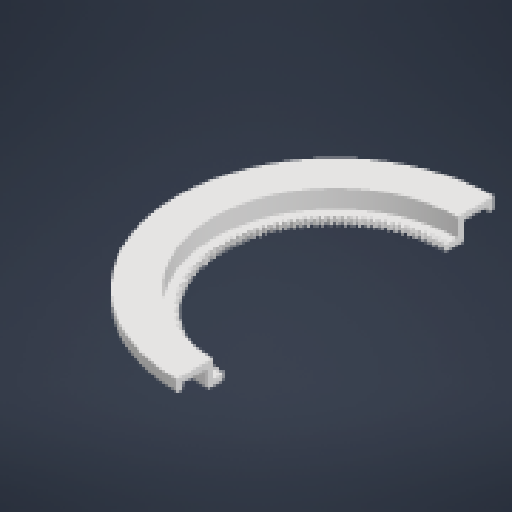
# Autodesk Inventor part: outerspinnerV3
Saved by Autodesk Inventor 2026 (Build 300175050, 175E)
## iProperties
Created: 2026-03-26
Part Number: outerspinnerV3
Material: Generic
Document SubType Name: Modeling
Designer: sniel
Density: 1 g/cm^3
Appearance: Default
Author: sniel
Autodesk Inventor part; units mm, degrees
ref_plane "YZ Plane" through (0, 0, 0) normal (1, 0, 0) x (0, 1, 0)
ref_plane "XZ Plane" through (0, 0, 0) normal (0, 1, 0) x (-1, 0, 0)
ref_plane "XY Plane" through (0, 0, 0) normal (0, 0, 1) x (1, 0, 0)
sketch "Sketch1" plane through (0, 0, 0) normal (0, 0, 1) x (1, 0, 0)
  line L0 (0, 0) -> (-100, 0)
  line L1 (-100, 0) -> (-100, 20)
  line L2 (-100, 20) -> (-130, 20)
  line L3 (-130, 20) -> (-130, 0)
  line L4 (-130, 0) -> (-100, 0)
  line L5 (-130, 0) -> (-125, 0)
  line L6 (-125, 0) -> (-125, 15)
  line L7 (-100, 0) -> (-105, 0)
  line L8 (-105, 0) -> (-105, 15)
  line L9 (-105, 15) -> (-125, 15)
  line L10 (0, -4) -> (0, 24) projected
  line L11 (-125, 15) -> (-125, 10)
  line L12 (-125, 10) -> (-130, 10)
  line L13 (-125, 15) -> (-115, 15)
  line L14 (-115, 15) -> (-117, 15)
  line L15 (-117, 15) -> (-117, 11)
  line L16 (-117, 11) -> (-113, 11)
  line L17 (-113, 11) -> (-113, 15)
  line L18 (-117, 15) -> (-119, 15)
  line L19 (-119, 15) -> (-119, 13)
  line L20 (-119, 13) -> (-117, 13)
  line L21 (-113, 15) -> (-111, 15)
  line L22 (-111, 15) -> (-111, 13)
  line L23 (-111, 13) -> (-113, 13)
  line L24 (-119, 15) -> (-118, 15)
  line L25 (-118, 15) -> (-118, 14)
  line L26 (-118, 14) -> (-119, 14)
  line L27 (-119, 14) -> (-119, 15)
  line L28 (-111, 15) -> (-112, 15)
  line L29 (-112, 15) -> (-112, 14)
  line L30 (-112, 14) -> (-111, 14)
  line L31 (-111, 14) -> (-111, 15)
  line L32 (-117, 13) -> (-119, 13)
  line L33 (-119, 13) -> (-119, 11)
  line L34 (-119, 11) -> (-117, 11)
  line L35 (-117, 11) -> (-117, 13)
  line L36 (-113, 13) -> (-111, 13)
  line L37 (-111, 13) -> (-111, 11)
  line L38 (-111, 11) -> (-113, 11)
  line L39 (-113, 11) -> (-113, 13)
  line L40 (-118, 14) -> (-112, 14)
  line L41 (-118, 14) -> (-118, 13)
  line L42 (-112, 14) -> (-112, 13)
  dimension "d0" = 100
  dimension "d1" = 20
  dimension "d2" = 30
  dimension "d3" = 5
  dimension "d4" = 15
  dimension "d5" = 5
  dimension "d7" = 5
  dimension "d8" = 2
  dimension "d9" = 4
  dimension "d10" = 4
  dimension "d11" = 2
  dimension "d12" = 2
  dimension "d13" = 2
  dimension "d22" = 1
  dimension "d23" = 1
  dimension "d24" = 1
  constraints: 84 end point, 16 perpendicular, 10 point on line, 8 parallel, 6 midpoint, 5 horizontal
  measures "d0" distance of L0.start L0.end
  measures "d1" distance of L0.end L1.end
  measures "d2" distance of L1.end L2.end
  measures "d3" distance of L3.end L5.end
  measures "d4" distance of L5.end L6.end
  measures "d5" distance of L0.end L7.end
  measures "d7" distance of L6.end L11.end
  measures "d8" distance of L13.end L14.end
  measures "d9" distance of L14.end L15.end
  measures "d10" distance of L15.end L16.end
  measures "d11" distance of L14.end L18.end
  measures "d12" distance of L18.end L19.end
  measures "d13" distance of L17.end L21.end
  measures "d22" distance of L24.end L25.end
  measures "d23" distance of L30.end L29.end
  measures "d24" distance of L29.end L28.end
revolve "Revolution1" add sketch "Sketch1" angle 360 about axis through (0, -10, 0) along (0, 1, 0) contours L4 L8 L9 L6 L12 L3 L2 L1 | L22 L30 L29 L9 | L9 L25 L26 L19
sketch "Sketch3" plane through (0, 0, 0) normal (0, -1, 0) x (1, 0, 0)
  circle A0 centre (0, 0) radius 102.0421
  arc A1 (-3.6556, 92.7167) -> (-4.7504, 92.6747) centre (-0.6449, 0) ccw
  arc A2 (-2.5377, 89.8188) -> (-3.6556, 92.7167) centre (-21.6763, 84.1004) ccw
  arc A3 (-2.4763, 89.6815) -> (-2.5377, 89.8188) centre (-14.4025, 84.4303) ccw
  arc A4 (-1.4378, 89.6967) -> (-2.4763, 89.6815) centre (-0.6449, 0) ccw
  arc A5 (-0.3693, 92.7652) -> (-1.4378, 89.6967) centre (17.8975, 84.684) ccw
  arc A6 (0.7262, 92.7554) -> (-0.3693, 92.7652) centre (-0.6449, 0) ccw
  arc A7 (1.7401, 89.6685) -> (0.7262, 92.7554) centre (-17.6812, 84.9998) ccw
  arc A8 (2.7781, 89.6349) -> (1.7401, 89.6685) centre (-0.6449, 0) ccw
  arc A9 (2.842, 89.7711) -> (2.7781, 89.6349) centre (14.6092, 84.1728) ccw
  arc A10 (4.0111, 92.6487) -> (2.842, 89.7711) centre (21.876, 83.7138) ccw
  arc A11 (5.105, 92.5872) -> (4.0111, 92.6487) centre (-0.6449, 0) ccw
  arc A12 (5.972, 89.4559) -> (5.105, 92.5872) centre (-13.6482, 85.7095) ccw
  arc A13 (7.028, 89.3715) -> (5.972, 89.4559) centre (-0.6449, 0) ccw
  arc A14 (8.3812, 92.3254) -> (7.028, 89.3715) centre (25.8042, 82.5569) ccw
  arc A15 (9.471, 92.2124) -> (8.3812, 92.3254) centre (-0.6449, 0) ccw
  arc A16 (10.1891, 89.0436) -> (9.471, 92.2124) centre (-9.5861, 86.2279) ccw
  arc A17 (11.24, 88.9094) -> (10.1891, 89.0436) centre (-0.6449, 0) ccw
  arc A18 (12.7312, 91.7962) -> (11.24, 88.9094) centre (29.6734, 81.2157) ccw
  arc A19 (13.8144, 91.6318) -> (12.7312, 91.7962) centre (-0.6449, 0) ccw
  arc A20 (14.382, 88.4326) -> (13.8144, 91.6318) centre (-5.504, 86.554) ccw
  arc A21 (15.4254, 88.249) -> (14.382, 88.4326) centre (-0.6449, 0) ccw
  arc A22 (17.0513, 91.0621) -> (15.4254, 88.249) centre (33.4749, 79.6934) ccw
  arc A23 (18.1255, 90.8467) -> (17.0513, 91.0621) centre (-0.6449, 0) ccw
  arc A24 (18.5414, 87.6243) -> (18.1255, 90.8467) centre (-1.4111, 86.6869) ccw
  arc A25 (19.575, 87.3916) -> (18.5414, 87.6243) centre (-0.6449, 0) ccw
  arc A26 (21.3319, 90.1248) -> (19.575, 87.3916) centre (37.2003, 77.9932) ccw
  arc A27 (22.3947, 89.8589) -> (21.3319, 90.1248) centre (-0.6449, 0) ccw
  arc A28 (22.658, 86.6205) -> (22.3947, 89.8589) centre (2.6835, 86.6263) ccw
  arc A29 (23.6794, 86.3392) -> (22.658, 86.6205) centre (-0.6449, 0) ccw
  arc A30 (25.5634, 88.9864) -> (23.6794, 86.3392) centre (40.8413, 76.1189) ccw
  arc A31 (26.6126, 88.6706) -> (25.5634, 88.9864) centre (-0.6449, 0) ccw
  arc A32 (26.7226, 85.4233) -> (26.6126, 88.6706) centre (6.7706, 86.3725) ccw
  arc A33 (27.7296, 85.0942) -> (26.7226, 85.4233) centre (-0.6449, 0) ccw
  arc A34 (29.7365, 87.6494) -> (27.7296, 85.0942) centre (44.3897, 74.0748) ccw
  arc A35 (30.7696, 87.2845) -> (29.7365, 87.6494) centre (-0.6449, 0) ccw
  arc A36 (30.7262, 84.0356) -> (30.7696, 87.2845) centre (10.8412, 85.9259) ccw
  arc A37 (31.7165, 83.6593) -> (30.7262, 84.0356) centre (-0.6449, 0) ccw
  arc A38 (33.8418, 86.1169) -> (31.7165, 83.6593) centre (47.8376, 71.8655) ccw
  arc A39 (34.8565, 85.7036) -> (33.8418, 86.1169) centre (-0.6449, 0) ccw
  arc A40 (34.6597, 82.4604) -> (34.8565, 85.7036) centre (14.8862, 85.2876) ccw
  arc A41 (35.6311, 82.0377) -> (34.6597, 82.4604) centre (-0.6449, 0) ccw
  arc A42 (37.8702, 84.3922) -> (35.6311, 82.0377) centre (51.1773, 69.4957) ccw
  arc A43 (38.8642, 83.9314) -> (37.8702, 84.3922) centre (-0.6449, 0) ccw
  arc A44 (38.5145, 80.7011) -> (38.8642, 83.9314) centre (18.8966, 84.459) ccw
  arc A45 (39.4648, 80.233) -> (38.5145, 80.7011) centre (-0.6449, 0) ccw
  arc A46 (41.8126, 82.4792) -> (39.4648, 80.233) centre (54.4014, 66.9709) ccw
  arc A47 (42.7837, 81.972) -> (41.8126, 82.4792) centre (-0.6449, 0) ccw
  arc A48 (42.2818, 78.7618) -> (42.7837, 81.972) centre (22.8633, 83.442) ccw
  arc A49 (43.209, 78.2494) -> (42.2818, 78.7618) centre (-0.6449, 0) ccw
  arc A50 (45.6602, 80.3821) -> (43.209, 78.2494) centre (57.5026, 64.2967) ccw
  arc A51 (46.6063, 79.8296) -> (45.6602, 80.3821) centre (-0.6449, 0) ccw
  arc A52 (45.9534, 76.6468) -> (46.6063, 79.8296) centre (26.7776, 82.2387) ccw
  arc A53 (46.8554, 76.0911) -> (45.9534, 76.6468) centre (-0.6449, 0) ccw
  arc A54 (49.4046, 78.1057) -> (46.8554, 76.0911) centre (60.4741, 61.4789) ccw
  arc A55 (50.3235, 77.5092) -> (49.4046, 78.1057) centre (-0.6449, 0) ccw
  arc A56 (49.521, 74.3607) -> (50.3235, 77.5092) centre (30.6306, 80.8519) ccw
  arc A57 (50.3958, 73.763) -> (49.521, 74.3607) centre (-0.6449, 0) ccw
  arc A58 (53.0372, 75.655) -> (50.3958, 73.763) centre (63.3092, 58.524) ccw
  arc A59 (53.927, 75.0157) -> (53.0372, 75.655) centre (-0.6449, 0) ccw
  arc A60 (52.9767, 71.9086) -> (53.927, 75.0157) centre (34.4139, 79.2848) ccw
  arc A61 (53.8222, 71.2703) -> (52.9767, 71.9086) centre (-0.6449, 0) ccw
  arc A62 (56.5501, 73.0355) -> (53.8222, 71.2703) centre (66.0017, 55.4385) ccw
  arc A63 (57.4087, 72.3549) -> (56.5501, 73.0355) centre (-0.6449, 0) ccw
  arc A64 (56.3127, 69.2962) -> (57.4087, 72.3549) centre (38.119, 77.5407) ccw
  arc A65 (57.1272, 68.6186) -> (56.3127, 69.2962) centre (-0.6449, 0) ccw
  arc A66 (59.9353, 70.253) -> (57.1272, 68.6186) centre (68.5453, 52.2293) ccw
  arc A67 (60.7608, 69.5326) -> (59.9353, 70.253) centre (-0.6449, 0) ccw
  arc A68 (59.5217, 66.5291) -> (60.7608, 69.5326) centre (41.7376, 75.6236) ccw
  arc A69 (60.3032, 65.8138) -> (59.5217, 66.5291) centre (-0.6449, 0) ccw
  arc A70 (63.1854, 67.3137) -> (60.3032, 65.8138) centre (70.9347, 48.9036) ccw
  arc A71 (63.976, 66.5552) -> (63.1854, 67.3137) centre (-0.6449, 0) ccw
  arc A72 (62.5963, 63.6135) -> (63.976, 66.5552) centre (45.2615, 73.5377) ccw
  arc A73 (63.3432, 62.8622) -> (62.5963, 63.6135) centre (-0.6449, 0) ccw
  arc A74 (66.2931, 64.2243) -> (63.3432, 62.8622) centre (73.1642, 45.4687) ccw
  arc A75 (67.0469, 63.4293) -> (66.2931, 64.2243) centre (-0.6449, 0) ccw
  arc A76 (65.5299, 60.556) -> (67.0469, 63.4293) centre (48.6831, 71.2878) ccw
  arc A77 (66.2404, 59.7702) -> (65.5299, 60.556) centre (-0.6449, 0) ccw
  arc A78 (69.2513, 60.9915) -> (66.2404, 59.7702) centre (75.2291, 41.9324) ccw
  arc A79 (69.9668, 60.1618) -> (69.2513, 60.9915) centre (-0.6449, 0) ccw
  arc A80 (68.3158, 57.3634) -> (69.9668, 60.1618) centre (51.9946, 68.8787) ccw
  arc A81 (68.9884, 56.5449) -> (68.3158, 57.3634) centre (-0.6449, 0) ccw
  arc A82 (72.0536, 57.6227) -> (68.9884, 56.5449) centre (77.1247, 38.3025) ccw
  arc A83 (72.7291, 56.7601) -> (72.0536, 57.6227) centre (-0.6449, 0) ccw
  arc A84 (70.9478, 54.0427) -> (72.7291, 56.7601) centre (55.1886, 66.316) ccw
  arc A85 (71.581, 53.1934) -> (70.9478, 54.0427) centre (-0.6449, 0) ccw
  arc A86 (74.6937, 54.1252) -> (71.581, 53.1934) centre (78.8468, 34.5872) ccw
  arc A87 (75.3277, 53.2317) -> (74.6937, 54.1252) centre (-0.6449, 0) ccw
  arc A88 (73.42, 50.6015) -> (75.3277, 53.2317) centre (58.2581, 63.6053) ccw
  arc A89 (74.0125, 49.7233) -> (73.42, 50.6015) centre (-0.6449, 0) ccw
  arc A90 (77.1657, 50.507) -> (74.0125, 49.7233) centre (80.3914, 30.7946) ccw
  arc A91 (77.7568, 49.5845) -> (77.1657, 50.507) centre (-0.6449, 0) ccw
  arc A92 (75.727, 47.0474) -> (77.7568, 49.5845) centre (61.1961, 60.7527) ccw
  arc A93 (76.2773, 46.1421) -> (75.727, 47.0474) centre (-0.6449, 0) ccw
  arc A94 (79.4641, 46.7761) -> (76.2773, 46.1421) centre (81.7553, 26.9334) ccw
  arc A95 (80.0109, 45.8267) -> (79.4641, 46.7761) centre (-0.6449, 0) ccw
  arc A96 (77.8636, 43.3883) -> (80.0109, 45.8267) centre (63.9961, 57.7645) ccw
  arc A97 (78.3706, 42.458) -> (77.8636, 43.3883) centre (-0.6449, 0) ccw
  arc A98 (81.5836, 42.9408) -> (78.3706, 42.458) centre (82.9352, 23.012) ccw
  arc A99 (82.0851, 41.9667) -> (81.5836, 42.9408) centre (-0.6449, 0) ccw
  arc A100 (79.825, 39.6323) -> (82.0851, 41.9667) centre (66.6519, 54.6474) ccw
  arc A101 (80.2875, 38.6792) -> (79.825, 39.6323) centre (-0.6449, 0) ccw
  arc A102 (83.5198, 39.0097) -> (80.2875, 38.6792) centre (83.9287, 19.0393) ccw
  arc A103 (83.9746, 38.013) -> (83.5198, 39.0097) centre (-0.6449, 0) ccw
  arc A104 (81.6068, 35.788) -> (83.9746, 38.013) centre (69.1575, 51.4084) ccw
  arc A105 (82.0238, 34.8141) -> (81.6068, 35.788) centre (-0.6449, 0) ccw
  arc A106 (85.2681, 34.9916) -> (82.0238, 34.8141) centre (84.7335, 15.0241) ccw
  arc A107 (85.6753, 33.9745) -> (85.2681, 34.9916) centre (-0.6449, 0) ccw
  arc A108 (83.2051, 31.8638) -> (85.6753, 33.9745) centre (71.5073, 48.0547) ccw
  arc A109 (83.5756, 30.8712) -> (83.2051, 31.8638) centre (-0.6449, 0) ccw
  arc A110 (86.8247, 30.8953) -> (83.5756, 30.8712) centre (85.3477, 10.9754) ccw
  arc A111 (87.1835, 29.8601) -> (86.8247, 30.8953) centre (-0.6449, 0) ccw
  arc A112 (84.6163, 27.8684) -> (87.1835, 29.8601) centre (73.6962, 44.5937) ccw
  arc A113 (84.9395, 26.8595) -> (84.6163, 27.8684) centre (-0.6449, 0) ccw
  arc A114 (88.1861, 26.7302) -> (84.9395, 26.8595) centre (85.7701, 6.9022) ccw
  arc A115 (88.4956, 25.6792) -> (88.1861, 26.7302) centre (-0.6449, 0) ccw
  arc A116 (85.8373, 23.8109) -> (88.4956, 25.6792) centre (75.7191, 41.0332) ccw
  arc A117 (86.1125, 22.7879) -> (85.8373, 23.8109) centre (-0.6449, 0) ccw
  arc A118 (89.3493, 22.5053) -> (86.1125, 22.7879) centre (85.9996, 2.8136) ccw
  arc A119 (89.6088, 21.4409) -> (89.3493, 22.5053) centre (-0.6449, 0) ccw
  arc A120 (86.8653, 19.7003) -> (89.6088, 21.4409) centre (77.5717, 37.3812) ccw
  arc A121 (87.0918, 18.6654) -> (86.8653, 19.7003) centre (-0.6449, 0) ccw
  arc A122 (90.3117, 18.2303) -> (87.0918, 18.6654) centre (86.0358, -1.2813) ccw
  arc A123 (90.5207, 17.1548) -> (90.3117, 18.2303) centre (-0.6449, 0) ccw
  arc A124 (87.698, 15.5457) -> (90.5207, 17.1548) centre (79.2498, 33.6458) ccw
  arc A125 (87.8754, 14.5013) -> (87.698, 15.5457) centre (-0.6449, 0) ccw
  arc A126 (91.0711, 13.9146) -> (87.8754, 14.5013) centre (85.8786, -5.3733) ccw
  arc A127 (91.2291, 12.8304) -> (91.0711, 13.9146) centre (-0.6449, 0) ccw
  arc A128 (88.3335, 11.3564) -> (91.2291, 12.8304) centre (80.7495, 29.8352) ccw
  arc A129 (88.4614, 10.3048) -> (88.3335, 11.3564) centre (-0.6449, 0) ccw
  arc A130 (91.6259, 9.5678) -> (88.4614, 10.3048) centre (85.5283, -9.4533) ccw
  arc A131 (91.7325, 8.4774) -> (91.6259, 9.5678) centre (-0.6449, 0) ccw
  arc A132 (88.7706, 7.1418) -> (91.7325, 8.4774) centre (82.0677, 25.9582) ccw
  arc A133 (88.8487, 6.0853) -> (88.7706, 7.1418) centre (-0.6449, 0) ccw
  arc A134 (91.9748, 5.1997) -> (88.8487, 6.0853) centre (84.9858, -13.5122) ccw
  arc A135 (92.0298, 4.1055) -> (91.9748, 5.1997) centre (-0.6449, 0) ccw
  arc A136 (89.0081, 2.9112) -> (92.0298, 4.1055) centre (83.2012, 22.0231) ccw
  arc A137 (89.0362, 1.8522) -> (89.0081, 2.9112) centre (-0.6449, 0) ccw
  arc A138 (92.117, 0.82) -> (89.0362, 1.8522) centre (84.2521, -17.541) ccw
  arc A139 (92.1202, -0.2756) -> (92.117, 0.82) centre (-0.6449, 0) ccw
  arc A140 (89.0455, -1.3258) -> (92.1202, -0.2756) centre (84.1477, 18.039) ccw
  arc A141 (89.0236, -2.385) -> (89.0455, -1.3258) centre (-0.6449, 0) ccw
  arc A142 (92.0523, -3.5615) -> (89.0236, -2.385) centre (83.329, -21.5307) ccw
  arc A143 (92.0037, -4.6561) -> (92.0523, -3.5615) centre (-0.6449, 0) ccw
  arc A144 (88.8828, -5.5599) -> (92.0037, -4.6561) centre (84.905, 14.0146) ccw
  arc A145 (88.8109, -6.6169) -> (88.8828, -5.5599) centre (-0.6449, 0) ccw
  arc A146 (91.7806, -7.9351) -> (88.8109, -6.6169) centre (82.2186, -25.4723) ccw
  arc A147 (91.6805, -9.0261) -> (91.7806, -7.9351) centre (-0.6449, 0) ccw
  arc A148 (88.5204, -9.7816) -> (91.6805, -9.0261) centre (85.4714, 9.9589) ccw
  arc A149 (88.3986, -10.834) -> (88.5204, -9.7816) centre (-0.6449, 0) ccw
  arc A150 (91.3028, -12.291) -> (88.3986, -10.834) centre (80.9232, -29.357) ccw
  arc A151 (91.1512, -13.3761) -> (91.3028, -12.291) centre (-0.6449, 0) ccw
  arc A152 (87.959, -13.9815) -> (91.1512, -13.3761) centre (85.8456, 5.881) ccw
  arc A153 (87.7877, -15.027) -> (87.959, -13.9815) centre (-0.6449, 0) ccw
  arc A154 (90.6198, -16.6195) -> (87.7877, -15.027) centre (79.4458, -33.1763) ccw
  arc A155 (90.4171, -17.6962) -> (90.6198, -16.6195) centre (-0.6449, 0) ccw
  arc A156 (87.1998, -18.1502) -> (90.4171, -17.6962) centre (86.0268, 1.79) ccw
  arc A157 (86.9794, -19.1864) -> (87.1998, -18.1502) centre (-0.6449, 0) ccw
  arc A158 (89.7331, -20.9109) -> (86.9794, -19.1864) centre (77.7898, -36.9215) ccw
  arc A159 (89.4798, -21.9768) -> (89.7331, -20.9109) centre (-0.6449, 0) ccw
  arc A160 (86.2447, -22.2783) -> (89.4798, -21.9768) centre (86.0147, -2.3051) ccw
  arc A161 (85.9755, -23.303) -> (86.2447, -22.2783) centre (-0.6449, 0) ccw
  arc A162 (88.6448, -25.1556) -> (85.9755, -23.303) centre (75.9587, -40.5844) ccw
  arc A163 (88.3414, -26.2084) -> (88.6448, -25.1556) centre (-0.6449, 0) ccw
  arc A164 (85.0957, -26.3568) -> (88.3414, -26.2084) centre (85.8091, -6.3949) ccw
  arc A165 (84.7784, -27.3676) -> (85.0957, -26.3568) centre (-0.6449, 0) ccw
  arc A166 (87.3572, -29.3442) -> (84.7784, -27.3676) centre (73.9566, -44.1566) ccw
  arc A167 (87.0045, -30.3815) -> (87.3572, -29.3442) centre (-0.6449, 0) ccw
  arc A168 (83.7553, -30.3764) -> (87.0045, -30.3815) centre (85.4107, -10.4706) ccw
  arc A169 (83.3907, -31.3711) -> (83.7553, -30.3764) centre (-0.6449, 0) ccw
  arc A170 (85.8732, -33.4673) -> (83.3907, -31.3711) centre (71.7881, -47.6304) ccw
  arc A171 (85.472, -34.4868) -> (85.8732, -33.4673) centre (-0.6449, 0) ccw
  arc A172 (82.2267, -34.3283) -> (85.472, -34.4868) centre (84.8202, -14.5228) ccw
  arc A173 (81.8155, -35.3046) -> (82.2267, -34.3283) centre (-0.6449, 0) ccw
  arc A174 (84.1962, -37.5157) -> (81.8155, -35.3046) centre (69.458, -50.9979) ccw
  arc A175 (83.7473, -38.5151) -> (84.1962, -37.5157) centre (-0.6449, 0) ccw
  arc A176 (80.5131, -38.2036) -> (83.7473, -38.5151) centre (84.039, -18.5426) ccw
  arc A177 (80.0562, -39.1594) -> (80.5131, -38.2036) centre (-0.6449, 0) ccw
  arc A178 (82.3299, -41.4804) -> (80.0562, -39.1594) centre (66.9714, -54.2515) ccw
  arc A179 (81.8342, -42.4575) -> (82.3299, -41.4804) centre (-0.6449, 0) ccw
  arc A180 (78.6184, -41.9936) -> (81.8342, -42.4575) centre (83.0689, -22.5211) ccw
  arc A181 (78.1169, -42.9268) -> (78.6184, -41.9936) centre (-0.6449, 0) ccw
  arc A182 (80.2785, -45.3526) -> (78.1169, -42.9268) centre (64.334, -57.3841) ccw
  arc A183 (79.7372, -46.3052) -> (80.2785, -45.3526) centre (-0.6449, 0) ccw
  arc A184 (76.5468, -45.6899) -> (79.7372, -46.3052) centre (81.9119, -26.4493) ccw
  arc A185 (76.0018, -46.5984) -> (76.5468, -45.6899) centre (-0.6449, 0) ccw
  arc A186 (78.0464, -49.1236) -> (76.0018, -46.5984) centre (61.5516, -60.3887) ccw
  arc A187 (77.4608, -50.0495) -> (78.0464, -49.1236) centre (-0.6449, 0) ccw
  arc A188 (74.303, -49.2843) -> (77.4608, -50.0495) centre (80.5708, -30.3185) ccw
  arc A189 (73.7157, -50.166) -> (74.303, -49.2843) centre (-0.6449, 0) ccw
  arc A190 (75.6388, -52.7849) -> (73.7157, -50.166) centre (58.6303, -63.2585) ccw
  arc A191 (75.0101, -53.6822) -> (75.6388, -52.7849) centre (-0.6449, 0) ccw
  arc A192 (71.892, -52.7686) -> (75.0101, -53.6822) centre (79.0484, -34.12) ccw
  arc A193 (71.2637, -53.6216) -> (71.892, -52.7686) centre (-0.6449, 0) ccw
  arc A194 (73.061, -56.3285) -> (71.2637, -53.6216) centre (55.5769, -65.9872) ccw
  arc A195 (72.3906, -57.195) -> (73.061, -56.3285) centre (-0.6449, 0) ccw
  arc A196 (69.3191, -56.1353) -> (72.3906, -57.195) centre (77.3482, -37.8454) ccw
  arc A197 (68.6512, -56.9577) -> (69.3191, -56.1353) centre (-0.6449, 0) ccw
  arc A198 (70.3186, -59.7463) -> (68.6512, -56.9577) centre (52.3979, -68.5686) ccw
  arc A199 (69.6081, -60.5803) -> (70.3186, -59.7463) centre (-0.6449, 0) ccw
  arc A200 (66.5901, -59.3767) -> (69.6081, -60.5803) centre (75.4739, -41.4864) ccw
  arc A201 (65.8841, -60.1666) -> (66.5901, -59.3767) centre (-0.6449, 0) ccw
  arc A202 (67.418, -63.0309) -> (65.8841, -60.1666) centre (49.1006, -70.997) ccw
  arc A203 (66.6688, -63.8303) -> (67.418, -63.0309) centre (-0.6449, 0) ccw
  arc A204 (63.711, -62.4855) -> (66.6688, -63.8303) centre (73.4298, -45.0348) ccw
  arc A205 (62.9686, -63.2412) -> (63.711, -62.4855) centre (-0.6449, 0) ccw
  arc A206 (64.3654, -66.1748) -> (62.9686, -63.2412) centre (45.6923, -73.267) ccw
  arc A207 (63.5794, -66.938) -> (64.3654, -66.1748) centre (-0.6449, 0) ccw
  arc A208 (60.6884, -65.455) -> (63.5794, -66.938) centre (71.2204, -48.4827) ccw
  arc A209 (59.9111, -66.1748) -> (60.6884, -65.455) centre (-0.6449, 0) ccw
  arc A210 (61.1678, -69.1711) -> (59.9111, -66.1748) centre (42.1806, -75.3735) ccw
  arc A211 (60.3466, -69.8963) -> (61.1678, -69.1711) centre (-0.6449, 0) ccw
  arc A212 (57.5289, -68.2784) -> (60.3466, -69.8963) centre (68.8507, -51.8224) ccw
  arc A213 (56.7184, -68.9607) -> (57.5289, -68.2784) centre (-0.6449, 0) ccw
  arc A214 (57.8323, -72.013) -> (56.7184, -68.9607) centre (38.5734, -77.3118) ccw
  arc A215 (56.9777, -72.6986) -> (57.8323, -72.013) centre (-0.6449, 0) ccw
  arc A216 (54.2396, -70.9495) -> (56.9777, -72.6986) centre (66.3259, -55.0464) ccw
  arc A217 (53.3978, -71.5927) -> (54.2396, -70.9495) centre (-0.6449, 0) ccw
  arc A218 (54.3663, -74.6942) -> (53.3978, -71.5927) centre (34.8786, -79.0777) ccw
  arc A219 (53.4803, -75.3386) -> (54.3663, -74.6942) centre (-0.6449, 0) ccw
  arc A220 (50.8278, -73.4622) -> (53.4803, -75.3386) centre (63.6516, -58.1477) ccw
  arc A221 (49.9566, -74.065) -> (50.8278, -73.4622) centre (-0.6449, 0) ccw
  arc A222 (50.7775, -77.2087) -> (49.9566, -74.065) centre (31.1046, -80.667) ccw
  arc A223 (49.8621, -77.8106) -> (50.7775, -77.2087) centre (-0.6449, 0) ccw
  arc A224 (47.3011, -75.811) -> (49.8621, -77.8106) centre (60.8339, -61.1192) ccw
  arc A225 (46.4025, -76.372) -> (47.3011, -75.811) centre (-0.6449, 0) ccw
  arc A226 (47.074, -79.551) -> (46.4025, -76.372) centre (27.2597, -82.0764) ccw
  arc A227 (46.1312, -80.109) -> (47.074, -79.551) centre (-0.6449, 0) ccw
  arc A228 (43.6675, -77.9906) -> (46.1312, -80.109) centre (57.879, -63.9543) ccw
  arc A229 (42.7433, -78.5085) -> (43.6675, -77.9906) centre (-0.6449, 0) ccw
  arc A230 (43.264, -81.7157) -> (42.7433, -78.5085) centre (23.3526, -83.3026) ccw
  arc A231 (42.2959, -82.2286) -> (43.264, -81.7157) centre (-0.6449, 0) ccw
  arc A232 (39.935, -79.9963) -> (42.2959, -82.2286) centre (54.7935, -66.6467) ccw
  arc A233 (38.9874, -80.4699) -> (39.935, -79.9963) centre (-0.6449, 0) ccw
  arc A234 (39.3561, -83.6981) -> (38.9874, -80.4699) centre (19.3919, -84.3429) ccw
  arc A235 (38.3648, -84.1647) -> (39.3561, -83.6981) centre (-0.6449, 0) ccw
  arc A236 (36.112, -81.8234) -> (38.3648, -84.1647) centre (51.5843, -69.1904) ccw
  arc A237 (35.1431, -82.2518) -> (36.112, -81.8234) centre (-0.6449, 0) ccw
  arc A238 (35.3589, -85.4937) -> (35.1431, -82.2518) centre (15.3865, -85.195) ccw
  arc A239 (34.3466, -85.913) -> (35.3589, -85.4937) centre (-0.6449, 0) ccw
  arc A240 (32.2069, -83.4679) -> (34.3466, -85.913) centre (48.2585, -71.5797) ccw
  arc A241 (31.2188, -83.8501) -> (32.2069, -83.4679) centre (-0.6449, 0) ccw
  arc A242 (31.2813, -87.0986) -> (31.2188, -83.8501) centre (11.3453, -85.857) ccw
  arc A243 (30.2504, -87.4696) -> (31.2813, -87.0986) centre (-0.6449, 0) ccw
  arc A244 (28.2285, -84.9262) -> (30.2504, -87.4696) centre (44.8237, -73.8093) ccw
  arc A245 (27.2235, -85.2613) -> (28.2285, -84.9262) centre (-0.6449, 0) ccw
  arc A246 (27.1325, -88.5091) -> (27.2235, -85.2613) centre (7.2774, -86.3275) ccw
  arc A247 (26.0852, -88.831) -> (27.1325, -88.5091) centre (-0.6449, 0) ccw
  arc A248 (24.1857, -86.195) -> (26.0852, -88.831) centre (41.2873, -75.8741) ccw
  arc A249 (23.166, -86.4822) -> (24.1857, -86.195) centre (-0.6449, 0) ccw
  arc A250 (22.9217, -89.7222) -> (23.166, -86.4822) centre (3.1918, -86.6053) ccw
  arc A251 (21.8604, -89.9942) -> (22.9217, -89.7222) centre (-0.6449, 0) ccw
  arc A252 (20.0875, -87.2714) -> (21.8604, -89.9942) centre (37.6574, -77.7697) ccw
  arc A253 (19.0554, -87.5102) -> (20.0875, -87.2714) centre (-0.6449, 0) ccw
  arc A254 (18.6583, -90.735) -> (19.0554, -87.5102) centre (-0.9024, -86.6899) ccw
  arc A255 (17.5854, -90.9566) -> (18.6583, -90.735) centre (-0.6449, 0) ccw
  arc A256 (15.943, -88.1531) -> (17.5854, -90.9566) centre (33.9421, -79.4917) ccw
  arc A257 (14.9008, -88.3429) -> (15.943, -88.1531) centre (-0.6449, 0) ccw
  arc A258 (14.3519, -91.5453) -> (14.9008, -88.3429) centre (-4.996, -86.581) ccw
  arc A259 (13.2697, -91.7161) -> (14.3519, -91.5453) centre (-0.6449, 0) ccw
  arc A260 (11.7615, -88.8381) -> (13.2697, -91.7161) centre (30.1495, -81.0364) ccw
  arc A261 (10.7115, -88.9785) -> (11.7615, -88.8381) centre (-0.6449, 0) ccw
  arc A262 (10.012, -92.1514) -> (10.7115, -88.9785) centre (-9.0799, -86.2789) ccw
  arc A263 (8.9229, -92.2708) -> (10.012, -92.1514) centre (-0.6449, 0) ccw
  arc A264 (7.5524, -89.3249) -> (8.9229, -92.2708) centre (26.2883, -82.4003) ccw
  arc A265 (6.4969, -89.4155) -> (7.5524, -89.3249) centre (-0.6449, 0) ccw
  arc A266 (5.6483, -92.5519) -> (6.4969, -89.4155) centre (-13.1449, -85.7843) ccw
  arc A267 (4.5548, -92.6197) -> (5.6483, -92.5519) centre (-0.6449, 0) ccw
  arc A268 (3.3249, -89.6123) -> (4.5548, -92.6197) centre (22.3669, -83.5802) ccw
  arc A269 (2.2663, -89.653) -> (3.3249, -89.6123) centre (-0.6449, 0) ccw
  arc A270 (1.2706, -92.7458) -> (2.2663, -89.653) centre (-17.1821, -85.0983) ccw
  arc A271 (0.1751, -92.762) -> (1.2706, -92.7458) centre (-0.6449, 0) ccw
  arc A272 (-0.9114, -89.6998) -> (0.1751, -92.762) centre (18.3942, -84.5737) ccw
  arc A273 (-1.9708, -89.6904) -> (-0.9114, -89.6998) centre (-0.6449, 0) ccw
  arc A274 (-3.1114, -92.7328) -> (-1.9708, -89.6904) centre (-21.1823, -84.2224) ccw
  arc A275 (-4.2065, -92.6972) -> (-3.1114, -92.7328) centre (-0.6449, 0) ccw
  arc A276 (-5.1471, -89.5872) -> (-4.2065, -92.6972) centre (14.379, -85.3784) ccw
  arc A277 (-6.2049, -89.5278) -> (-5.1471, -89.5872) centre (-0.6449, 0) ccw
  arc A278 (-7.4879, -92.5128) -> (-6.2049, -89.5278) centre (-25.1368, -83.1586) ccw
  arc A279 (-8.5801, -92.4256) -> (-7.4879, -92.5128) centre (-0.6449, 0) ccw
  arc A280 (-9.3728, -89.2746) -> (-8.5801, -92.4256) centre (10.3303, -85.9927) ccw
  arc A281 (-10.4266, -89.1653) -> (-9.3728, -89.2746) centre (-0.6449, 0) ccw
  arc A282 (-11.8492, -92.0865) -> (-10.4266, -89.1653) centre (-29.0366, -81.9092) ccw
  arc A283 (-12.936, -91.9477) -> (-11.8492, -92.0865) centre (-0.6449, 0) ccw
  arc A284 (-13.579, -88.7628) -> (-12.936, -91.9477) centre (6.2571, -86.415) ccw
  arc A285 (-14.6264, -88.6039) -> (-13.579, -88.7628) centre (-0.6449, 0) ccw
  arc A286 (-16.1854, -91.4546) -> (-14.6264, -88.6039) centre (-32.873, -80.477) ccw
  arc A287 (-17.2644, -91.2647) -> (-16.1854, -91.4546) centre (-0.6449, 0) ccw
  arc A288 (-17.7564, -88.053) -> (-17.2644, -91.2647) centre (2.1685, -86.6446) ccw
  arc A289 (-18.7951, -87.8448) -> (-17.7564, -88.053) centre (-0.6449, 0) ccw
  arc A290 (-20.487, -90.6187) -> (-18.7951, -87.8448) centre (-36.6375, -78.8653) ccw
  arc A291 (-21.5558, -90.378) -> (-20.487, -90.6187) centre (-0.6449, 0) ccw
  arc A292 (-21.8955, -87.1467) -> (-21.5558, -90.378) centre (-1.9264, -86.6808) ccw
  arc A293 (-22.9233, -86.8896) -> (-21.8955, -87.1467) centre (-0.6449, 0) ccw
  arc A294 (-24.7442, -89.5806) -> (-22.9233, -86.8896) centre (-40.3217, -77.0775) ccw
  arc A295 (-25.8005, -89.2897) -> (-24.7442, -89.5806) centre (-0.6449, 0) ccw
  arc A296 (-25.9873, -86.0459) -> (-25.8005, -89.2897) centre (-6.0184, -86.5235) ccw
  arc A297 (-27.0017, -85.7406) -> (-25.9873, -86.0459) centre (-0.6449, 0) ccw
  arc A298 (-28.9477, -88.3425) -> (-27.0017, -85.7406) centre (-43.9174, -75.1178) ccw
  arc A299 (-29.9891, -88.0021) -> (-28.9477, -88.3425) centre (-0.6449, 0) ccw
  arc A300 (-30.0225, -84.7531) -> (-29.9891, -88.0021) centre (-10.0984, -86.1733) ccw
  arc A301 (-31.0214, -84.4003) -> (-30.0225, -84.7531) centre (-0.6449, 0) ccw
  arc A302 (-33.0881, -86.9074) -> (-31.0214, -84.4003) centre (-47.4165, -72.9905) ccw
  arc A303 (-34.1122, -86.5182) -> (-33.0881, -86.9074) centre (-0.6449, 0) ccw
  arc A304 (-33.9921, -83.2712) -> (-34.1122, -86.5182) centre (-14.1573, -85.6307) ccw
  arc A305 (-34.9732, -82.8716) -> (-33.9921, -83.2712) centre (-0.6449, 0) ccw
  arc A306 (-37.156, -85.2783) -> (-34.9732, -82.8716) centre (-50.8113, -70.7003) ccw
  arc A307 (-38.1606, -84.8412) -> (-37.156, -85.2783) centre (-0.6449, 0) ccw
  arc A308 (-37.8873, -81.6035) -> (-38.1606, -84.8412) centre (-18.1861, -84.897) ccw
  arc A309 (-38.8485, -81.158) -> (-37.8873, -81.6035) centre (-0.6449, 0) ccw
  arc A310 (-41.1425, -83.459) -> (-38.8485, -81.158) centre (-54.0941, -68.2524) ccw
  arc A311 (-42.1254, -82.9749) -> (-41.1425, -83.459) centre (-0.6449, 0) ccw
  arc A312 (-41.6995, -79.7537) -> (-42.1254, -82.9749) centre (-22.1758, -83.9739) ccw
  arc A313 (-42.6385, -79.2633) -> (-41.6995, -79.7537) centre (-0.6449, 0) ccw
  arc A314 (-45.0386, -81.4534) -> (-42.6385, -79.2633) centre (-57.2577, -65.6521) ccw
  arc A315 (-45.9975, -80.9234) -> (-45.0386, -81.4534) centre (-0.6449, 0) ccw
  arc A316 (-45.42, -77.726) -> (-45.9975, -80.9234) centre (-26.1174, -82.8635) ccw
  arc A317 (-46.3348, -77.1918) -> (-45.42, -77.726) centre (-0.6449, 0) ccw
  arc A318 (-48.8357, -79.266) -> (-46.3348, -77.1918) centre (-60.2949, -62.9053) ccw
  arc A319 (-49.7685, -78.6914) -> (-48.8357, -79.266) centre (-0.6449, 0) ccw
  arc A320 (-49.0406, -75.5248) -> (-49.7685, -78.6914) centre (-30.0021, -81.5681) ccw
  arc A321 (-49.9292, -74.9479) -> (-49.0406, -75.5248) centre (-0.6449, 0) ccw
  arc A322 (-52.5252, -76.9018) -> (-49.9292, -74.9479) centre (-63.199, -60.0182) ccw
  arc A323 (-53.4298, -76.2837) -> (-52.5252, -76.9018) centre (-0.6449, 0) ccw
  arc A324 (-52.5532, -73.1551) -> (-53.4298, -76.2837) centre (-33.8214, -80.0907) ccw
  arc A325 (-53.4136, -72.5369) -> (-52.5532, -73.1551) centre (-0.6449, 0) ccw
  arc A326 (-56.099, -74.366) -> (-53.4136, -72.5369) centre (-65.9635, -56.9972) ccw
  arc A327 (-56.9734, -73.7059) -> (-56.099, -74.366) centre (-0.6449, 0) ccw
  arc A328 (-55.95, -70.6221) -> (-56.9734, -73.7059) centre (-37.5666, -78.4346) ccw
  arc A329 (-56.7802, -69.964) -> (-55.95, -70.6221) centre (-0.6449, 0) ccw
  arc A330 (-59.549, -71.6642) -> (-56.7802, -69.964) centre (-68.5823, -53.849) ccw
  arc A331 (-60.3913, -70.9636) -> (-59.549, -71.6642) centre (-0.6449, 0) ccw
  arc A332 (-59.2234, -67.9316) -> (-60.3913, -70.9636) centre (-41.2294, -76.6035) ccw
  arc A333 (-60.0216, -67.235) -> (-59.2234, -67.9316) centre (-0.6449, 0) ccw
  arc A334 (-62.8676, -68.8026) -> (-60.0216, -67.235) centre (-71.0495, -50.5806) ccw
  arc A335 (-63.6758, -68.0629) -> (-62.8676, -68.8026) centre (-0.6449, 0) ccw
  arc A336 (-62.3661, -65.0894) -> (-63.6758, -68.0629) centre (-44.8017, -74.6014) ccw
  arc A337 (-63.1305, -64.356) -> (-62.3661, -65.0894) centre (-0.6449, 0) ccw
  arc A338 (-66.0473, -65.7874) -> (-63.1305, -64.356) centre (-73.3596, -47.1993) ccw
  arc A339 (-66.8197, -65.0104) -> (-66.0473, -65.7874) centre (-0.6449, 0) ccw
  arc A340 (-65.371, -62.1021) -> (-66.8197, -65.0104) centre (-48.2755, -72.4329) ccw
  arc A341 (-66.0999, -61.3333) -> (-65.371, -62.1021) centre (-0.6449, 0) ccw
  arc A342 (-69.0811, -62.6254) -> (-66.0999, -61.3333) centre (-75.5074, -43.7128) ccw
  arc A343 (-69.816, -61.8128) -> (-69.0811, -62.6254) centre (-0.6449, 0) ccw
  arc A344 (-68.2315, -58.9761) -> (-69.816, -61.8128) centre (-51.6429, -70.1028) ccw
  arc A345 (-68.9233, -58.1738) -> (-68.2315, -58.9761) centre (-0.6449, 0) ccw
  arc A346 (-71.9622, -59.3237) -> (-68.9233, -58.1738) centre (-77.4882, -40.1287) ccw
  arc A347 (-72.6579, -58.4772) -> (-71.9622, -59.3237) centre (-0.6449, 0) ccw
  arc A348 (-70.9412, -55.7186) -> (-72.6579, -58.4772) centre (-54.8966, -67.6162) ccw
  arc A349 (-71.5944, -54.8845) -> (-70.9412, -55.7186) centre (-0.6449, 0) ccw
  arc A350 (-74.6842, -55.8895) -> (-71.5944, -54.8845) centre (-79.2975, -36.455) ccw
  arc A351 (-75.3391, -55.0112) -> (-74.6842, -55.8895) centre (-0.6449, 0) ccw
  arc A352 (-73.4941, -52.3367) -> (-75.3391, -55.0112) centre (-58.0292, -64.9788) ccw
  arc A353 (-74.1071, -51.4727) -> (-73.4941, -52.3367) centre (-0.6449, 0) ccw
  arc A354 (-77.2409, -52.3307) -> (-74.1071, -51.4727) centre (-80.9313, -32.7) ccw
  arc A355 (-77.8536, -51.4225) -> (-77.2409, -52.3307) centre (-0.6449, 0) ccw
  arc A356 (-75.8844, -48.8381) -> (-77.8536, -51.4225) centre (-61.0338, -62.1964) ccw
  arc A357 (-76.4559, -47.9461) -> (-75.8844, -48.8381) centre (-0.6449, 0) ccw
  arc A358 (-79.6268, -48.6551) -> (-76.4559, -47.9461) centre (-82.386, -28.872) ccw
  arc A359 (-80.1959, -47.719) -> (-79.6268, -48.6551) centre (-0.6449, 0) ccw
  arc A360 (-78.1068, -45.2304) -> (-80.1959, -47.719) centre (-63.9036, -59.2751) ccw
  arc A361 (-78.6356, -44.3124) -> (-78.1068, -45.2304) centre (-0.6449, 0) ccw
  arc A362 (-81.8364, -44.871) -> (-78.6356, -44.3124) centre (-83.6583, -24.9797) ccw
  arc A363 (-82.3606, -43.909) -> (-81.8364, -44.871) centre (-0.6449, 0) ccw
  arc A364 (-80.1563, -41.5219) -> (-82.3606, -43.909) centre (-66.6322, -56.2216) ccw
  arc A365 (-80.6412, -40.5799) -> (-80.1563, -41.5219) centre (-0.6449, 0) ccw
  arc A366 (-83.8648, -40.9867) -> (-80.6412, -40.5799) centre (-84.7453, -21.0315) ccw
  arc A367 (-84.343, -40.001) -> (-83.8648, -40.9867) centre (-0.6449, 0) ccw
  arc A368 (-82.0285, -37.7207) -> (-84.343, -40.001) centre (-69.2136, -53.0427) ccw
  arc A369 (-82.4683, -36.7569) -> (-82.0285, -37.7207) centre (-0.6449, 0) ccw
  arc A370 (-85.7075, -37.011) -> (-82.4683, -36.7569) centre (-85.6447, -17.0365) ccw
  arc A371 (-86.1387, -36.0038) -> (-85.7075, -37.011) centre (-0.6449, 0) ccw
  arc A372 (-83.719, -33.8353) -> (-86.1387, -36.0038) centre (-71.6421, -49.7454) ccw
  arc A373 (-84.1128, -32.8518) -> (-83.719, -33.8353) centre (-0.6449, 0) ccw
  arc A374 (-87.3604, -32.9526) -> (-84.1128, -32.8518) centre (-86.3544, -13.0034) ccw
  arc A375 (-87.7435, -31.9262) -> (-87.3604, -32.9526) centre (-0.6449, 0) ccw
  arc A376 (-85.2242, -29.8744) -> (-87.7435, -31.9262) centre (-73.912, -46.3371) ccw
  arc A377 (-85.5711, -28.8734) -> (-85.2242, -29.8744) centre (-0.6449, 0) ccw
  arc A378 (-88.8198, -28.8208) -> (-85.5711, -28.8734) centre (-86.8728, -8.9413) ccw
  arc A379 (-89.1541, -27.7774) -> (-88.8198, -28.8208) centre (-0.6449, 0) ccw
  arc A380 (-86.5406, -25.8469) -> (-89.1541, -27.7774) centre (-76.0185, -42.8254) ccw
  arc A381 (-86.8399, -24.8306) -> (-86.5406, -25.8469) centre (-0.6449, 0) ccw
  arc A382 (-90.0825, -24.6246) -> (-86.8399, -24.8306) centre (-87.1989, -4.8593) ccw
  arc A383 (-90.3671, -23.5666) -> (-90.0825, -24.6246) centre (-0.6449, 0) ccw
  arc A384 (-87.6654, -21.7617) -> (-90.3671, -23.5666) centre (-77.9569, -39.2182) ccw
  arc A385 (-87.9163, -20.7324) -> (-87.6654, -21.7617) centre (-0.6449, 0) ccw
  arc A386 (-91.1456, -20.3735) -> (-87.9163, -20.7324) centre (-87.3318, -0.7664) ccw
  arc A387 (-91.3799, -19.3033) -> (-91.1456, -20.3735) centre (-0.6449, 0) ccw
  arc A388 (-88.596, -17.6279) -> (-91.3799, -19.3033) centre (-79.7227, -35.5234) ccw
  arc A389 (-88.798, -16.588) -> (-88.596, -17.6279) centre (-0.6449, 0) ccw
  arc A390 (-92.0068, -16.0769) -> (-88.798, -16.588) centre (-87.2713, 3.3282) ccw
  arc A391 (-92.1903, -14.9968) -> (-92.0068, -16.0769) centre (-0.6449, 0) ccw
  arc A392 (-89.3303, -13.4548) -> (-92.1903, -14.9968) centre (-81.312, -31.7494) ccw
  arc A393 (-89.483, -12.4065) -> (-89.3303, -13.4548) centre (-0.6449, 0) ccw
  arc A394 (-92.6641, -11.7445) -> (-89.483, -12.4065) centre (-87.0174, 7.4154) ccw
  arc A395 (-92.7963, -10.6569) -> (-92.6641, -11.7445) centre (-0.6449, 0) ccw
  arc A396 (-89.8668, -9.2517) -> (-92.7963, -10.6569) centre (-82.7213, -27.9045) ccw
  arc A397 (-89.9698, -8.1973) -> (-89.8668, -9.2517) centre (-0.6449, 0) ccw
  arc A398 (-93.116, -7.3858) -> (-89.9698, -8.1973) centre (-86.5709, 11.486) ccw
  arc A399 (-93.1968, -6.2932) -> (-93.116, -7.3858) centre (-0.6449, 0) ccw
  arc A400 (-90.2041, -5.0279) -> (-93.1968, -6.2932) centre (-83.9475, -23.9973) ccw
  arc A401 (-90.2573, -3.9698) -> (-90.2041, -5.0279) centre (-0.6449, 0) ccw
  arc A402 (-93.3616, -3.0107) -> (-90.2573, -3.9698) centre (-85.9326, 15.531) ccw
  arc A403 (-93.3907, -1.9155) -> (-93.3616, -3.0107) centre (-0.6449, 0) ccw
  arc A404 (-90.3417, -0.7929) -> (-93.3907, -1.9155) centre (-84.9879, -20.0366) ccw
  arc A405 (-90.3448, 0.2665) -> (-90.3417, -0.7929) centre (-0.6449, 0) ccw
  arc A406 (-93.4004, 1.3711) -> (-90.3448, 0.2665) centre (-85.104, 19.5413) ccw
  arc A407 (-93.3777, 2.4665) -> (-93.4004, 1.3711) centre (-0.6449, 0) ccw
  arc A408 (-90.279, 3.4438) -> (-93.3777, 2.4665) centre (-85.84, -16.0312) ccw
  arc A409 (-90.2321, 4.5022) -> (-90.279, 3.4438) centre (-0.6449, 0) ccw
  arc A410 (-93.2321, 5.7499) -> (-90.2321, 4.5022) centre (-84.0869, 23.508) ccw
  arc A411 (-93.1578, 6.843) -> (-93.2321, 5.7499) centre (-0.6449, 0) ccw
  arc A412 (-90.0164, 7.6729) -> (-93.1578, 6.843) centre (-86.502, -11.9901) ccw
  arc A413 (-89.9195, 8.7279) -> (-90.0164, 7.6729) centre (-0.6449, 0) ccw
  arc A414 (-92.8573, 10.1159) -> (-89.9195, 8.7279) centre (-82.8837, 27.4223) ccw
  arc A415 (-92.7314, 11.2042) -> (-92.8573, 10.1159) centre (-0.6449, 0) ccw
  arc A416 (-89.5543, 11.8849) -> (-92.7314, 11.2042) centre (-86.9724, -7.9221) ccw
  arc A417 (-89.4078, 12.9341) -> (-89.5543, 11.8849) centre (-0.6449, 0) ccw
  arc A418 (-92.2767, 14.4593) -> (-89.4078, 12.9341) centre (-81.4969, 31.2754) ccw
  arc A419 (-92.0995, 15.5405) -> (-92.2767, 14.4593) centre (-0.6449, 0) ccw
  arc A420 (-88.8939, 16.0703) -> (-92.0995, 15.5405) centre (-87.2502, -3.8365) ccw
  arc A421 (-88.6979, 17.1114) -> (-88.8939, 16.0703) centre (-0.6449, 0) ccw
  arc A422 (-91.4916, 18.7704) -> (-88.6979, 17.1114) centre (-79.9298, 35.0587) ccw
  arc A423 (-91.2636, 19.842) -> (-91.4916, 18.7704) centre (-0.6449, 0) ccw
  arc A424 (-88.0365, 20.2199) -> (-91.2636, 19.842) centre (-87.3348, 0.2576) ccw
  arc A425 (-87.7916, 21.2506) -> (-88.0365, 20.2199) centre (-0.6449, 0) ccw
  arc A426 (-90.5039, 23.0397) -> (-87.7916, 21.2506) centre (-78.1857, 38.7638) ccw
  arc A427 (-90.2255, 24.0993) -> (-90.5039, 23.0397) centre (-0.6449, 0) ccw
  arc A428 (-86.9841, 24.3244) -> (-90.2255, 24.0993) centre (-87.2259, 4.3512) ccw
  arc A429 (-86.6908, 25.3423) -> (-86.9841, 24.3244) centre (-0.6449, 0) ccw
  arc A430 (-89.3156, 27.2575) -> (-86.6908, 25.3423) centre (-76.2686, 42.3823) ccw
  arc A431 (-88.9875, 28.3028) -> (-89.3156, 27.2575) centre (-0.6449, 0) ccw
  arc A432 (-85.7391, 28.3745) -> (-88.9875, 28.3028) centre (-86.9238, 8.4351) ccw
  arc A433 (-85.3981, 29.3775) -> (-85.7391, 28.3745) centre (-0.6449, 0) ccw
  arc A434 (-87.9294, 31.4145) -> (-85.3981, 29.3775) centre (-74.1827, 45.9063) ccw
  arc A435 (-87.5523, 32.4432) -> (-87.9294, 31.4145) centre (-0.6449, 0) ccw
  arc A436 (-84.3042, 32.3614) -> (-87.5523, 32.4432) centre (-86.4292, 12.5002) ccw
  arc A437 (-83.9162, 33.3472) -> (-84.3042, 32.3614) centre (-0.6449, 0) ccw
  arc A438 (-86.3485, 35.5014) -> (-83.9162, 33.3472) centre (-71.9328, 49.3279) ccw
  arc A439 (-85.9232, 36.5111) -> (-86.3485, 35.5014) centre (-0.6449, 0) ccw
  arc A440 (-82.6826, 36.2761) -> (-85.9232, 36.5111) centre (-85.7432, 16.5373) ccw
  arc A441 (-82.2485, 37.2424) -> (-82.6826, 36.2761) centre (-0.6449, 0) ccw
  arc A442 (-84.5763, 39.5091) -> (-82.2485, 37.2424) centre (-69.5238, 52.6394) ccw
  arc A443 (-84.1039, 40.4976) -> (-84.5763, 39.5091) centre (-0.6449, 0) ccw
  arc A444 (-80.878, 40.1098) -> (-84.1039, 40.4976) centre (-84.8673, 20.5376) ccw
  arc A445 (-80.3987, 41.0545) -> (-80.878, 40.1098) centre (-0.6449, 0) ccw
  arc A446 (-82.6169, 43.4286) -> (-80.3987, 41.0545) centre (-66.9611, 55.8334) ccw
  arc A447 (-82.0983, 44.3937) -> (-82.6169, 43.4286) centre (-0.6449, 0) ccw
  arc A448 (-78.8943, 43.854) -> (-82.0983, 44.3937) centre (-83.8034, 24.492) ccw
  arc A449 (-78.3709, 44.7751) -> (-78.8943, 43.854) centre (-0.6449, 0) ccw
  arc A450 (-80.4746, 47.2513) -> (-78.3709, 44.7751) centre (-64.2504, 58.9029) ccw
  arc A451 (-79.9109, 48.1908) -> (-80.4746, 47.2513) centre (-0.6449, 0) ccw
  arc A452 (-76.736, 47.5003) -> (-79.9109, 48.1908) centre (-82.554, 28.3918) ccw
  arc A453 (-76.1697, 48.3957) -> (-76.736, 47.5003) centre (-0.6449, 0) ccw
  arc A454 (-78.1541, 50.9685) -> (-76.1697, 48.3957) centre (-61.3977, 61.8409) ccw
  arc A455 (-77.5467, 51.8803) -> (-78.1541, 50.9685) centre (-0.6449, 0) ccw
  arc A456 (-74.4079, 51.0407) -> (-77.5467, 51.8803) centre (-81.1219, 32.2283) ccw
  arc A457 (-73.8, 51.9083) -> (-74.4079, 51.0407) centre (-0.6449, 0) ccw
  arc A458 (-75.6607, 54.5719) -> (-73.8, 51.9083) centre (-58.4096, 64.6409) ccw
  arc A459 (-75.0109, 55.4541) -> (-75.6607, 54.5719) centre (-0.6449, 0) ccw
  arc A460 (-71.9153, 54.4672) -> (-75.0109, 55.4541) centre (-79.5101, 35.9928) ccw
  arc A461 (-71.267, 55.3051) -> (-71.9153, 54.4672) centre (-0.6449, 0) ccw
  arc A462 (-72.9998, 58.0536) -> (-71.267, 55.3051) centre (-55.2925, 67.2967) ccw
  arc A463 (-72.3092, 58.9041) -> (-72.9998, 58.0536) centre (-0.6449, 0) ccw
  arc A464 (-69.2636, 57.7721) -> (-72.3092, 58.9041) centre (-77.7224, 39.677) ccw
  arc A465 (-68.5765, 58.5785) -> (-69.2636, 57.7721) centre (-0.6449, 0) ccw
  arc A466 (-70.1776, 61.4058) -> (-68.5765, 58.5785) centre (-52.0535, 69.8023) ccw
  arc A467 (-69.4475, 62.2227) -> (-70.1776, 61.4058) centre (-0.6449, 0) ccw
  arc A468 (-66.4588, 60.9481) -> (-69.4475, 62.2227) centre (-75.7627, 43.2727) ccw
  arc A469 (-65.7344, 61.7211) -> (-66.4588, 60.9481) centre (-0.6449, 0) ccw
  arc A470 (-67.2001, 64.6209) -> (-65.7344, 61.7211) centre (-48.6997, 72.1522) ccw
  arc A471 (-66.4323, 65.4024) -> (-67.2001, 64.6209) centre (-0.6449, 0) ccw
  arc A472 (-63.5071, 63.9881) -> (-66.4323, 65.4024) centre (-73.6353, 46.7718) ccw
  arc A473 (-62.747, 64.7261) -> (-63.5071, 63.9881) centre (-0.6449, 0) ccw
  arc A474 (-64.0742, 67.6918) -> (-62.747, 64.7261) centre (-45.2388, 74.341) ccw
  arc A475 (-63.2703, 68.4362) -> (-64.0742, 67.6918) centre (-0.6449, 0) ccw
  arc A476 (-60.4152, 66.8854) -> (-63.2703, 68.4362) centre (-71.3451, 50.1665) ccw
  arc A477 (-59.6211, 67.5866) -> (-60.4152, 66.8854) centre (-0.6449, 0) ccw
  arc A478 (-60.8067, 70.6117) -> (-59.6211, 67.5866) centre (-41.6783, 76.364) ccw
  arc A479 (-59.9686, 71.3173) -> (-60.8067, 70.6117) centre (-0.6449, 0) ccw
  arc A480 (-57.1898, 69.6334) -> (-59.9686, 71.3173) centre (-68.8972, 53.4493) ccw
  arc A481 (-56.3635, 70.2963) -> (-57.1898, 69.6334) centre (-0.6449, 0) ccw
  arc A482 (-57.405, 73.374) -> (-56.3635, 70.2963) centre (-38.0263, 78.2166) ccw
  arc A483 (-56.5345, 74.0393) -> (-57.405, 73.374) centre (-0.6449, 0) ccw
  arc A484 (-53.8384, 72.226) -> (-56.5345, 74.0393) centre (-66.2969, 56.6129) ccw
  arc A485 (-52.9817, 72.8492) -> (-53.8384, 72.226) centre (-0.6449, 0) ccw
  arc A486 (-53.8766, 75.9726) -> (-52.9817, 72.8492) centre (-34.2909, 79.8946) ccw
  arc A487 (-52.9757, 76.596) -> (-53.8766, 75.9726) centre (-0.6449, 0) ccw
  arc A488 (-50.3682, 74.6574) -> (-52.9757, 76.596) centre (-63.5501, 59.6501) ccw
  arc A489 (-49.483, 75.2395) -> (-50.3682, 74.6574) centre (-0.6449, 0) ccw
  arc A490 (-50.2295, 78.4017) -> (-49.483, 75.2395) centre (-30.4803, 81.3944) ccw
  arc A491 (-49.3001, 78.9818) -> (-50.2295, 78.4017) centre (-0.6449, 0) ccw
  arc A492 (-46.7871, 76.9223) -> (-49.3001, 78.9818) centre (-60.663, 62.5542) ccw
  arc A493 (-45.8754, 77.4619) -> (-46.7871, 76.9223) centre (-0.6449, 0) ccw
  arc A494 (-46.4717, 80.6558) -> (-45.8754, 77.4619) centre (-26.6032, 82.7125) ccw
  arc A495 (-45.5159, 81.1914) -> (-46.4717, 80.6558) centre (-0.6449, 0) ccw
  arc A496 (-43.103, 79.0155) -> (-45.5159, 81.1914) centre (-57.642, 65.3187) ccw
  arc A497 (-42.1668, 79.5114) -> (-43.103, 79.0155) centre (-0.6449, 0) ccw
  arc A498 (-42.6116, 82.73) -> (-42.1668, 79.5114) centre (-22.6682, 83.8461) ccw
  arc A499 (-41.6316, 83.2198) -> (-42.6116, 82.73) centre (-0.6449, 0) ccw
  arc A500 (-39.3241, 80.9324) -> (-41.6316, 83.2198) centre (-54.4937, 67.9375) ccw
  arc A501 (-38.3656, 81.3836) -> (-39.3241, 80.9324) centre (-0.6449, 0) ccw
  arc A502 (-38.6579, 84.6195) -> (-38.3656, 81.3836) centre (-18.6841, 84.7926) ccw
  arc A503 (-37.6559, 85.0626) -> (-38.6579, 84.6195) centre (-0.6449, 0) ccw
  arc A504 (-35.459, 82.6687) -> (-37.6559, 85.0626) centre (-51.2254, 70.4047) ccw
  arc A505 (-34.4802, 83.0741) -> (-35.459, 82.6687) centre (-0.6449, 0) ccw
  arc A506 (-34.6194, 86.3203) -> (-34.4802, 83.0741) centre (-14.6597, 85.5499) ccw
  arc A507 (-33.5976, 86.7155) -> (-34.6194, 86.3203) centre (-0.6449, 0) ccw
  arc A508 (-31.5162, 84.2205) -> (-33.5976, 86.7155) centre (-47.8441, 72.7148) ccw
  arc A509 (-30.5194, 84.5793) -> (-31.5162, 84.2205) centre (-0.6449, 0) ccw
  arc A510 (-30.5051, 87.8284) -> (-30.5194, 84.5793) centre (-10.604, 86.1163) ccw
  arc A511 (-29.4657, 88.1749) -> (-30.5051, 87.8284) centre (-0.6449, 0) ccw
  arc A512 (-27.5045, 85.5844) -> (-29.4657, 88.1749) centre (-44.3575, 74.8626) ccw
  arc A513 (-26.4918, 85.8957) -> (-27.5045, 85.5844) centre (-0.6449, 0) ccw
  arc A514 (-26.3241, 89.1405) -> (-26.4918, 85.8957) centre (-6.5261, 86.4905) ccw
  arc A515 (-25.2696, 89.4376) -> (-26.3241, 89.1405) centre (-0.6449, 0) ccw
  arc A516 (-23.4328, 86.7574) -> (-25.2696, 89.4376) centre (-40.7734, 76.8434) ccw
  arc A517 (-22.4066, 87.0205) -> (-23.4328, 86.7574) centre (-0.6449, 0) ccw
  arc A518 (-22.0859, 90.2538) -> (-22.4066, 87.0205) centre (-2.4351, 86.6718) ccw
  arc A519 (-21.0184, 90.5007) -> (-22.0859, 90.2538) centre (-0.6449, 0) ccw
  arc A520 (-19.3103, 87.7367) -> (-21.0184, 90.5007) centre (-37.0998, 78.6527) ccw
  arc A521 (-18.2728, 87.9511) -> (-19.3103, 87.7367) centre (-0.6449, 0) ccw
  arc A522 (-17.7997, 91.1656) -> (-18.2728, 87.9511) centre (1.66, 86.6596) ccw
  arc A523 (-16.7219, 91.3618) -> (-17.7997, 91.1656) centre (-0.6449, 0) ccw
  arc A524 (-15.1462, 88.5203) -> (-16.7219, 91.3618) centre (-33.3448, 80.2865) ccw
  arc A525 (-14.0997, 88.6854) -> (-15.1462, 88.5203) centre (-0.6449, 0) ccw
  arc A526 (-13.4754, 91.874) -> (-14.0997, 88.6854) centre (5.7498, 86.4541) ccw
  arc A527 (-12.3894, 92.0191) -> (-13.4754, 91.874) centre (-0.6449, 0) ccw
  arc A528 (-10.9497, 89.1064) -> (-12.3894, 92.0191) centre (-29.5168, 81.7411) ccw
  arc A529 (-9.8966, 89.2219) -> (-10.9497, 89.1064) centre (-0.6449, 0) ccw
  arc A530 (-9.1224, 92.3774) -> (-9.8966, 89.2219) centre (9.8255, 86.0556) ccw
  arc A531 (-8.0308, 92.4711) -> (-9.1224, 92.3774) centre (-0.6449, 0) ccw
  arc A532 (-6.7302, 89.4936) -> (-8.0308, 92.4711) centre (-25.6244, 83.0134) ccw
  arc A533 (-5.6728, 89.5592) -> (-6.7302, 89.4936) centre (-0.6449, 0) ccw
  arc A534 (-4.7504, 92.6747) -> (-5.6728, 89.5592) centre (13.8777, 85.4651) ccw
  point P0 (0, 0)
  constraints: 1068 point on circle, 535 centre point
extrude "Extrusion2" add sketch "Sketch3" against normal blind 5
fillet "Fillet1" radius 2 3 edges at (105, 0, 0) (130, 10, 0) (125, 10, 0)
sketch "Sketch4" plane through (0, 0, 0) normal (1, 0, 0) x (0, 1, 0)
  line L0 (-23.5802, 140.97) -> (43.5802, 140.97)
  line L1 (43.5802, 140.97) -> (43.5802, -140.97)
  line L2 (43.5802, -140.97) -> (-23.5802, -140.97)
  line L3 (-23.5802, -140.97) -> (-23.5802, 140.97)
  line L4 (10, -130) -> (10, 130) projected
  line L5 (-23.5802, 140.97) -> (43.5802, -140.97) construction
  line L6 (43.5802, 140.97) -> (-23.5802, -140.97) construction
  point P0 (0, 0)
  point P1 (10, 0)
  constraints: 12 end point, 3 midpoint, 2 parallel, 1 horizontal, 1 perpendicular
extrude "Extrusion3" cut sketch "Sketch4" along normal blind 144.7
sketch "Sketch5" plane through (0, 0, 0) normal (0, 0, 1) x (1, 0, 0)
  line L0 (161.925, 66.675) -> (-184.15, 66.675)
  line L1 (-184.15, 66.675) -> (-184.15, -36.5125)
  line L2 (-184.15, -36.5125) -> (161.925, -36.5125)
  line L3 (161.925, -36.5125) -> (161.925, 66.675)
  point P0 (0, 0)
  constraints: 8 end point, 2 parallel, 1 horizontal, 1 perpendicular
extrude "Extrusion4" [suppressed]
body "Solid1"
